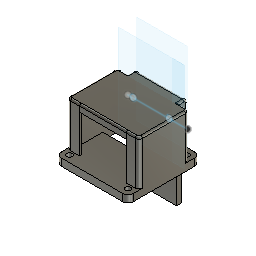
Optical Cube mk1 v4 (Autodesk Fusion 360 design; units mm, degrees)
Autodesk Fusion 360 part; units mm, degrees
note: some values were not read from the file. Set by a fixed rule: which sketch regions a step uses.
sketch "Sketch1" plane through (0, 0, 0) normal (0, 0, 1) x (1, 0, 0)
  line L0 (17, -20) -> (-17, -20)
  line L1 (-20, -17) -> (-20, 17)
  line L2 (-17, 20) -> (17, 20)
  line L3 (20, 17) -> (20, -17)
  line L4 (20, -20) -> (-20, 20) construction
  line L5 (-20, -20) -> (20, 20) construction
  arc A0 (-17, 20) -> (-20, 17) centre (-17, 17) ccw
  arc A1 (20, 17) -> (17, 20) centre (17, 17) ccw
  arc A2 (-20, -17) -> (-17, -20) centre (-17, -17) ccw
  arc A3 (17, -20) -> (20, -17) centre (17, -17) ccw
  dimension "d1" = 40
  dimension "d2" = 40
  dimension "d7" = 3
  dimension "d8" = 3
  dimension "d9" = 3
  dimension "d10" = 3
  constraint horizontal L0
  constraint perpendicular L0 L1
  constraint parallel L0 L2
  constraint parallel L1 L3
  constraint coincident L4 origin
  constraint coincident L5 origin
  constraint coincident L4.end L2
  constraint coincident L4.end L1
  constraint tangent L2 A0
  constraint tangent L1 A0
  constraint coincident L5.end L2
  constraint coincident L5.end L3
  constraint tangent L2 A1
  constraint tangent L3 A1
  constraint coincident L5.start L0
  constraint coincident L5.start L1
  constraint tangent L0 A2
  constraint tangent L1 A2
  constraint coincident L4.start L3
  constraint coincident L4.start L0
  constraint tangent L3 A3
  constraint tangent L0 A3
  measures "d1" distance of L4.end L5.end
  measures "d2" distance of L5.start L4.end
  measures "d7" radius of A0
  measures "d8" radius of A1
  measures "d9" radius of A2
  measures "d10" radius of A3
extrude "Extrude1" add sketch "Sketch1" along normal blind 4
sketch "Sketch3" plane through (0, 0, 4) normal (0, 0, 1) x (-1, 0, 0)
  arc A0 (20, 17) -> (17, 20) centre (17, 17) ccw
  line L0 (17, 20) -> (-17, 20)
  arc A1 (-17, 20) -> (-20, 17) centre (-17, 17) ccw
  line L1 (-20, 17) -> (-20, -17)
  arc A2 (-20, -17) -> (-17, -20) centre (-17, -17) ccw
  line L2 (-17, -20) -> (17, -20)
  arc A3 (17, -20) -> (20, -17) centre (17, -17) ccw
  line L3 (20, -17) -> (20, 17)
  circle A4 centre (16.2929, -16.2929) radius 1.5
  circle A5 centre (-16.2929, -16.2929) radius 1.5
  circle A6 centre (16.2929, 16.2929) radius 1.5
  circle A7 centre (-16.2929, 16.2929) radius 1.5
  line L4 (13.9939, -20) -> (13.9939, -14)
  line L5 (13.9939, -14) -> (20, -14)
  line L6 (20, 13.9693) -> (13.9939, 13.9693)
  line L7 (13.9939, 13.9693) -> (13.9939, 20)
  line L8 (-14.051, 20) -> (-14.051, 13.9693)
  line L9 (-14.051, 13.9693) -> (-20, 13.9693)
  line L10 (-20, -14) -> (-14.051, -14)
  line L11 (-14.051, -14) -> (-14.051, -20)
  line L12 (13.9939, -18.9303) -> (-14.051, -18.9303)
  line L13 (13.9939, 18.9046) -> (-14.051, 18.9046)
  line L14 (18.9336, 13.9693) -> (18.9336, -14)
  line L15 (-19, -14) -> (-19, 13.9693)
  line L16 (18.9336, -12.9942) -> (13, -12.9942)
  line L17 (13, -12.9942) -> (13, -18.9303)
  line L18 (17.9849, -12.9942) -> (17.9849, 13)
  line L19 (17.9849, 13) -> (13, 13)
  line L20 (13, 13) -> (13, 18)
  line L21 (13, 18) -> (-13, 18)
  line L22 (-13, 18) -> (-13, 13)
  line L23 (-13, 13) -> (-18, 13)
  line L24 (-18, 13) -> (-18, -13)
  line L25 (-18, -13) -> (-13, -13)
  line L26 (-13, -13) -> (-13, -18)
  line L27 (-13, -18) -> (13, -18)
  dimension "d13" = 3
  dimension "d15" = 3
  dimension "d17" = 3
  dimension "d19" = 3
  constraint coincident L2 L4.start
  constraint perpendicular L2 L4
  constraint coincident L3 L5.end
  constraint perpendicular L3 L5
  constraint coincident L3 L6.start
  constraint perpendicular L3 L6
  constraint coincident L0 L7.end
  constraint perpendicular L0 L7
  constraint coincident L0 L8.start
  constraint perpendicular L0 L8
  constraint coincident L1 L9.end
  constraint perpendicular L1 L9
  constraint coincident L1 L10.start
  constraint perpendicular L1 L10
  constraint coincident L2 L11.end
  constraint perpendicular L2 L11
  constraint coincident L4 L12.start
  constraint coincident L11 L12.end
  constraint perpendicular L11 L12
  constraint coincident L7 L13.start
  constraint coincident L8 L13.end
  constraint perpendicular L8 L13
  constraint coincident L6 L14.start
  constraint coincident L5 L14.end
  constraint perpendicular L5 L14
  constraint coincident L10 L15.start
  constraint coincident L9 L15.end
  constraint perpendicular L9 L15
  constraint coincident L14 L16.start
  constraint perpendicular L14 L16
  constraint coincident L12 L17.end
  constraint perpendicular L12 L17
  constraint coincident L16 L18.start
  constraint perpendicular L16 L18
  constraint perpendicular L18 L19
  constraint perpendicular L13 L20
  constraint perpendicular L8 L21
  constraint perpendicular L21 L22
  constraint perpendicular L22 L23
  constraint perpendicular L9 L24
  constraint perpendicular L24 L25
  constraint perpendicular L25 L26
  constraint coincident L17 L27.end
  constraint perpendicular L17 L27
  measures "d13" diameter of A4
  measures "d15" diameter of A5
  measures "d17" diameter of A6
  measures "d19" diameter of A7
extrude "Extrude2" add sketch "Sketch3" along normal blind 50 contours L6 L7 L8 L9 L10 L11 L12 L13 L14 L15 L16 L17 L18 L19 L20 L21 L22 L23 L24 L25 L26 L27 | L4 L5 L12 L14 L16 L17
extrude "Extrude4" cut sketch "Sketch3" against normal blind 42 contours A5
extrude "Extrude5" cut sketch "Sketch3" against normal blind 14 contours A4
extrude "Extrude6" cut sketch "Sketch3" against normal blind 15 contours A6
extrude "Extrude7" cut sketch "Sketch3" against normal blind 15 contours A7
extrude "Extrude8" add sketch "Sketch3" along normal blind 50 contours L16 L17 L18 L19 L20 L21 L22 L23 L24 L25 L26 L27
sketch "Sketch4" plane through (0, 0, 0) normal (0, 0, -1) x (1, 0, 0)
  circle A0 centre (16.2929, 16.2929) radius 1.5
  circle A1 centre (-16.2929, 16.2929) radius 1.5
  circle A2 centre (-16.2929, -16.2929) radius 1.5
  circle A3 centre (16.2929, -16.2929) radius 1.5
  arc A4 (-17, 20) -> (-20, 17) centre (-17, 17) ccw
  line L0 (-20, 17) -> (-20, -17)
  arc A5 (-20, -17) -> (-17, -20) centre (-17, -17) ccw
  line L1 (-17, -20) -> (17, -20)
  arc A6 (17, -20) -> (20, -17) centre (17, -17) ccw
  line L2 (20, -17) -> (20, 17)
  arc A7 (20, 17) -> (17, 20) centre (17, 17) ccw
  line L3 (17, 20) -> (-17, 20)
  line L4 (12, -18) -> (12, -13)
  line L5 (12, -13) -> (18, -13)
  line L6 (18, -13) -> (18, 13)
  line L7 (18, 13) -> (13, 13)
  line L8 (13, 13) -> (13, 18)
  line L9 (13, 18) -> (-13, 18)
  line L10 (-13, 18) -> (-13, 13)
  line L11 (-13, 13) -> (-18, 13)
  line L12 (-18, 13) -> (-18, -13)
  line L13 (-18, -13) -> (-13, -13)
  line L14 (-13, -13) -> (-13, -18)
  line L15 (-13, -18) -> (12, -18)
  constraint vertical L4
  constraint perpendicular L4 L5
  constraint perpendicular L5 L6
  constraint perpendicular L6 L7
  constraint perpendicular L7 L8
  constraint perpendicular L8 L9
  constraint perpendicular L9 L10
  constraint perpendicular L10 L11
  constraint perpendicular L11 L12
  constraint perpendicular L0 L13
  constraint perpendicular L13 L14
  constraint perpendicular L4 L15
extrude "Extrude9" cut sketch "Sketch4" against normal blind 50 contours L4 L5 L6 L7 L8 L9 L10 L11 L12 L13 L14 L15
sketch "Sketch5" plane through (-18, 0, 0) normal (1, 0, 0) x (0, 1, 0)
  line L0 (-13, 0) -> (13, 0)
  line L1 (13, 0) -> (13, 50)
  line L2 (13, 50) -> (-13, 50)
  line L3 (-13, 50) -> (-13, 0)
  line L4 (13, 0) -> (11, 0)
  line L5 (11, 0) -> (11, 50)
  line L6 (11, 50) -> (13, 50)
  line L7 (13, 50) -> (13, 0)
  dimension "d36" = 2
  dimension "d37" = 50
  constraint horizontal L4
  constraint vertical L5
  constraint horizontal L6
  constraint vertical L7
  constraint coincident L0.end L1.start
  measures "d36" distance of L0.end L4.end
  measures "d37" distance of L0.end L1.end
extrude "Extrude10" cut sketch "Sketch5" against normal blind 0.3 contours L0 L1 L2 L4 L5 L6 L7
sketch "Sketch6" plane through (18, 0, 0) normal (-1, 0, 0) x (0, -1, 0)
  line L0 (-13, 0) -> (13, 0)
  line L1 (13, 0) -> (13, 50)
  line L2 (13, 50) -> (-13, 50)
  line L3 (-13, 50) -> (-13, 0)
  line L4 (-13, 0) -> (-11, 0)
  line L5 (-11, 0) -> (-11, 50)
  line L6 (-11, 50) -> (-13, 50)
  line L7 (-13, 50) -> (-13, 0)
  dimension "d40" = 2
  dimension "d41" = 50
  constraint horizontal L4
  constraint vertical L5
  constraint horizontal L6
  constraint vertical L7
  constraint coincident L0.start L3.end
  measures "d40" distance of L0.start L4.end
  measures "d41" distance of L0.start L2.end
extrude "Extrude11" cut sketch "Sketch6" against normal blind 0.3 contours L0 L2 L3 L4 L5 L6 L7
sketch "Sketch7" plane through (-13.9939, 0, 0) normal (-1, 0, 0) x (0, -1, 0)
  line L0 (-18.9303, 4) -> (-14, 4)
  line L1 (-14, 4) -> (-14, 54)
  line L2 (-14, 54) -> (-18.9303, 54)
  line L3 (-18.9303, 54) -> (-18.9303, 4)
  line L4 (-18.9303, 54) -> (-14, 54)
  line L5 (-14, 54) -> (-14, 14)
  line L6 (-14, 14) -> (-18.9303, 14)
  line L7 (-18.9303, 14) -> (-18.9303, 54)
  constraint horizontal L4
  constraint vertical L5
  constraint horizontal L6
  constraint vertical L7
  constraint coincident L1 L5.end
  constraint coincident L2.end L3.start
extrude "Extrude12" add sketch "Sketch7" against normal blind 28 contours L1 L2 L3 L4 L5 L6 L7
sketch "Sketch9" plane through (0, 18.9303, 0) normal (0, 1, 0) x (-1, 0, 0)
  line L0 (-14.051, 4) -> (13.9939, 4)
  line L1 (13.9939, 4) -> (13.9939, 54)
  line L2 (13.9939, 54) -> (-14.051, 54)
  line L3 (-14.051, 54) -> (-14.051, 4)
  line L4 (18.9939, 14) -> (-14.051, 14)
  constraint coincident L3 L4.end
  constraint perpendicular L3 L4
sketch "Sketch11" plane through (14.051, 0, 0) normal (1, 0, 0) x (0, 1, 0)
  line L0 (14, 4) -> (18.9303, 4)
  line L1 (18.9303, 4) -> (18.9303, 54)
  line L2 (18.9303, 54) -> (14, 54)
  line L3 (14, 54) -> (14, 4)
  line L4 (14, 54) -> (18.9303, 54)
  line L5 (18.9303, 54) -> (18.9303, 13.913)
  line L6 (18.9303, 13.913) -> (14, 13.913)
  line L7 (14, 13.913) -> (14, 54)
  constraint horizontal L4
  constraint vertical L5
  constraint horizontal L6
  constraint vertical L7
  constraint coincident L1 L5.end
  constraint coincident L2.end L3.start
extrude "Extrude13" add sketch "Sketch11" along normal blind 5 contours L1 L2 L3 L4 L5 L6 L7
sketch "Sketch12" plane through (0, -18, 0) normal (0, 1, 0) x (-1, 0, 0)
  line L0 (-13, 0) -> (13, 0)
  line L1 (13, 0) -> (13, 50)
  line L2 (13, 50) -> (-13, 50)
  line L3 (-13, 50) -> (-13, 0)
  line L4 (-13, 50) -> (13, 50)
  line L5 (13, 50) -> (13, -6)
  line L6 (13, -6) -> (-13, -6)
  line L7 (-13, -6) -> (-13, 50)
  constraint horizontal L4
  constraint vertical L5
  constraint horizontal L6
  constraint vertical L7
  constraint coincident L2.end L3.start
extrude "Extrude14" cut sketch "Sketch12" against normal blind 13 contours L0 L1 L2 L3 L4 L5 L7
sketch "Sketch13" plane through (0, 13, 0) normal (0, -1, 0) x (1, 0, 0)
  line L0 (12, 0) -> (18.3, 0)
  line L1 (18.3, 0) -> (18.3, 50)
  line L2 (18.3, 50) -> (12, 50)
  line L3 (12, 50) -> (12, 0)
extrude "Extrude15" add 1 faces at (-13, 15, 4.6667) along direction (1, 0, 0) blind 26
extrude "Extrude16" cut 1 faces at (19.051, 15.6434, 40.6377) along direction (-1, 0, 0) blind 5
sketch "Sketch14" plane through (14.051, 0, 0) normal (1, 0, 0) x (0, 1, 0)
  line L0 (14, 54) -> (14, 4)
  line L1 (14, 4) -> (18.9303, 4)
  line L2 (18.9303, 4) -> (18.9303, 54)
  line L3 (18.9303, 54) -> (14, 54)
  line L4 (18.9303, 54) -> (14, 54)
  line L5 (14, 54) -> (14, 35)
  line L6 (14, 35) -> (18.9303, 35)
  line L7 (18.9303, 35) -> (18.9303, 54)
  constraint horizontal L4
  constraint vertical L5
  constraint horizontal L6
  constraint vertical L7
  constraint coincident L0 L5.end
  constraint coincident L2.end L3.start
extrude "Extrude17" add sketch "Sketch14" along normal blind 5 contours L0 L2 L3 L4 L5 L6 L7
sketch "Sketch15" plane through (-13.9939, 0, 0) normal (-1, 0, 0) x (0, -1, 0)
  line L0 (-18.9303, 54) -> (-18.9303, 4)
  line L1 (-18.9303, 4) -> (-14, 4)
  line L2 (-14, 4) -> (-14, 54)
  line L3 (-14, 54) -> (-18.9303, 54)
  line L4 (-18.9303, 54) -> (-14, 54)
  line L5 (-14, 54) -> (-14, 35)
  line L6 (-14, 35) -> (-18.9303, 35)
  line L7 (-18.9303, 35) -> (-18.9303, 54)
  constraint horizontal L4
  constraint vertical L5
  constraint horizontal L6
  constraint vertical L7
  constraint coincident L2 L5.end
  constraint coincident L0.start L3.end
extrude "Extrude18" add sketch "Sketch15" along normal blind 5 contours L0 L2 L3 L4 L5 L6 L7
sketch "Sketch16" plane through (0, 13, 0) normal (0, -1, 0) x (1, 0, 0)
  line L0 (-18.3, 0) -> (18.3, 0)
  line L1 (18.3, 0) -> (18.3, 50)
  line L2 (18.3, 50) -> (-18.3, 50)
  line L3 (-18.3, 50) -> (-18.3, 0)
  circle A0 centre (9.8744, 20.0869) radius 1.5
  circle A1 centre (-10.1256, 20.0869) radius 1.5
  dimension "d61" = 3
  dimension "d62" = 3
  dimension "d93" = 20
  measures "d61" diameter of A0
  measures "d62" diameter of A1
  measures "d93" distance of A0.centre A1.centre
extrude "Extrude19" cut sketch "Sketch16" against normal blind 12 contours A0 | A1
extrude "Extrude20" add 1 faces at (-13.9939, -15.6144, 37.3333) along direction (-1, 0, 0) blind 5
extrude "Extrude21" add 1 faces at (14.051, -17.2595, 37.3333) along direction (1, 0, 0) blind 5
sketch "Sketch17" plane through (19.051, 0, 0) normal (1, 0, 0) x (0, 1, 0)
  line L0 (-18.9046, 4) -> (-13.9693, 4)
  line L1 (-13.9693, 4) -> (-13.9693, 54)
  line L2 (-13.9693, 54) -> (-18.9046, 54)
  line L3 (-18.9046, 54) -> (-18.9046, 4)
  line L4 (-18.9046, 34.9752) -> (-13.9693, 34.9752)
  line L5 (-13.9693, 34.9752) -> (-13.9693, 4)
  line L6 (-13.9693, 4) -> (-18.9046, 4)
  line L7 (-18.9046, 4) -> (-18.9046, 34.9752)
  constraint horizontal L4
  constraint vertical L5
  constraint horizontal L6
  constraint vertical L7
  constraint coincident L0.end L1.start
  constraint coincident L3 L4.start
extrude "Extrude22" cut sketch "Sketch17" against normal blind 8 contours L0 L1 L3 L4 L5 L6 L7
sketch "Sketch18" plane through (-18.9939, 0, 0) normal (-1, 0, 0) x (0, -1, 0)
  line L0 (13.9693, 4) -> (18.9046, 4)
  line L1 (18.9046, 4) -> (18.9046, 54)
  line L2 (18.9046, 54) -> (13.9693, 54)
  line L3 (13.9693, 54) -> (13.9693, 4)
  line L4 (18.9046, 4) -> (13.9693, 4)
  line L5 (13.9693, 4) -> (13.9693, 35.0999)
  line L6 (13.9693, 35.0999) -> (18.9046, 35.0999)
  line L7 (18.9046, 35.0999) -> (18.9046, 4)
  constraint horizontal L4
  constraint vertical L5
  constraint horizontal L6
  constraint vertical L7
  constraint coincident L3 L5.end
  constraint coincident L0.end L1.start
extrude "Extrude23" cut sketch "Sketch18" against normal blind 6 contours L0 L1 L3 L4 L5 L6 L7
sketch "Sketch19" plane through (13, 0, 0) normal (-1, 0, 0) x (0, -1, 0)
  line L0 (13.9693, 34.9752) -> (18.9046, 34.9752)
  line L1 (18.9046, 34.9752) -> (18.9046, 50)
  line L2 (18.9046, 50) -> (13, 50)
  line L3 (13, 50) -> (13, 0)
  line L4 (13, 0) -> (20, 0)
  line L5 (20, 0) -> (20, 4)
  line L6 (20, 4) -> (13.9693, 4)
  line L7 (13.9693, 4) -> (13.9693, 34.9752)
  line L8 (20, 0) -> (13, 0)
  line L9 (13, 0) -> (13, 4)
  line L10 (13, 4) -> (20, 4)
  line L11 (20, 4) -> (20, 0)
  constraint horizontal L8
  constraint vertical L9
  constraint horizontal L10
  constraint vertical L11
  constraint coincident L3 L9.end
  constraint coincident L4.end L5.start
extrude "Extrude24" add sketch "Sketch19" along normal blind 26 contours L3 L4 L5 L6 L8 L9 L10 L11
sketch "Sketch20" plane through (0, -13, 0) normal (0, 1, 0) x (-1, 0, 0)
  line L0 (-18, 0) -> (18, 0)
  line L1 (18, 0) -> (18, 50)
  line L2 (18, 50) -> (13, 50)
  line L3 (13, 50) -> (13, 4)
  line L4 (13, 4) -> (-13, 4)
  line L5 (-13, 4) -> (-13, 50)
  line L6 (-13, 50) -> (-18, 50)
  line L7 (-18, 50) -> (-18, 0)
  line L8 (18, 0) -> (-18, 0)
  line L9 (-18, 0) -> (-18, 4)
  line L10 (-18, 4) -> (18, 4)
  line L11 (18, 4) -> (18, 0)
  constraint horizontal L8
  constraint vertical L9
  constraint horizontal L10
  constraint vertical L11
  constraint coincident L7 L9.end
  constraint coincident L0.end L1.start
extrude "Extrude25" add sketch "Sketch20" along normal blind 17 contours L0 L1 L4 L7 L8 L9 L10 L11
sketch "Sketch21" plane through (0, 4, 0) normal (0, 1, 0) x (-1, 0, 0)
  line L0 (18, 4) -> (-18, 4)
  line L1 (-18, 4) -> (-18, 0)
  line L2 (-18, 0) -> (18, 0)
  line L3 (18, 0) -> (18, 4)
  line L4 (-18, 4) -> (-13, 4)
  line L5 (-13, 4) -> (-13, 0)
  line L6 (-13, 0) -> (-18, 0)
  line L7 (-18, 0) -> (-18, 4)
  line L8 (18, 4) -> (13, 4)
  line L9 (13, 4) -> (13, 0)
  line L10 (13, 0) -> (18, 0)
  line L11 (18, 0) -> (18, 4)
  constraint horizontal L4
  constraint vertical L5
  constraint horizontal L6
  constraint vertical L7
  constraint coincident L2 L5.end
  constraint coincident L0.end L1.start
  constraint horizontal L8
  constraint vertical L9
  constraint horizontal L10
  constraint vertical L11
  constraint coincident L2 L9.end
  constraint coincident L0.start L3.end
extrude "Extrude26" add sketch "Sketch21" along normal blind 7 contours L0 L2 L3 L8 L9 L10 L11 | L0 L1 L2 L4 L5 L6 L7
extrude "Extrude27" add 1 faces at (13, 8.6667, 2.6667) along direction (-1, 0, 0) blind 5
extrude "Extrude28" add 1 faces at (-13, 8.6667, 2.6667) along direction (1, 0, 0) blind 5
extrude "Extrude29" cut 1 faces at (8, 8.6667, 2.6667) along direction (1, 0, 0) blind 10
extrude "Extrude30" cut 1 faces at (-8, 8.6667, 2.6667) along direction (-1, 0, 0) blind 10
extrude "Extrude31" add 1 faces at (19, 4.6769, 24.6584) along direction (1, 0, 0) blind 1
extrude "Extrude32" add 1 faces at (-18.9336, -4.6462, 24.7) along direction (-1, 0, 0) blind 1
move_face "OffsetFaces1" offset 3 1 faces at (-4.3333, 3, 50)
move_face "OffsetFaces2" offset -1 1 faces at (-4.3333, 3, 47)
extrude "Extrude33" add 1 faces at (-18.9939, 17.2869, 41.3333) along direction (-1, 0, 0) blind 1
extrude "Extrude34" add 1 faces at (-18.9939, -15.6144, 41.3999) along direction (-1, 0, 0) blind 1
extrude "Extrude35" add 1 faces at (19.051, -17.2595, 41.3168) along direction (1, 0, 0) blind 1
extrude "Extrude36" add 1 faces at (19.051, 15.6434, 47.6667) along direction (1, 0, 0) blind 1
fillet "Fillet1" radius 3 1 edges at (20.051, 18.9303, 44.5)
fillet "Fillet2" radius 3 1 edges at (-19.9939, 18.9303, 44.5)
fillet "Fillet3" radius 3 1 edges at (-19.9939, -18.9046, 44.5499)
fillet "Fillet4" radius 3 1 edges at (20.051, -18.9046, 44.4876)
move_face "OffsetFaces3" offset 8 1 faces at (-4.3333, 3, 48)
move_face "OffsetFaces4" offset -10 1 faces at (6.6888, -4.6462, 54)
sketch "Sketch22" plane through (0, 0, 0) normal (0, 0, -1) x (1, 0, 0)
  line L0 (-18, -11) -> (-18, -4)
  line L1 (-18, -4) -> (18, -4)
  line L2 (18, -4) -> (18, -11)
  line L3 (18, -11) -> (18.3, -11)
  line L4 (18.3, -11) -> (18.3, -13)
  line L5 (18.3, -13) -> (-18.3, -13)
  line L6 (-18.3, -13) -> (-18.3, -11)
  line L7 (-18.3, -11) -> (-18, -11)
  circle A0 centre (16.2929, 16.2929) radius 1.5
  circle A1 centre (-16.2929, 16.2929) radius 1.5
  circle A2 centre (-16.2929, -16.2929) radius 1.5
  circle A3 centre (16.2929, -16.2929) radius 1.5
  line L8 (17, 20) -> (-17, 20)
  arc A4 (-17, 20) -> (-20, 17) centre (-17, 17) ccw
  line L9 (-20, 17) -> (-20, -17)
  arc A5 (-20, -17) -> (-17, -20) centre (-17, -17) ccw
  line L10 (-17, -20) -> (17, -20)
  arc A6 (17, -20) -> (20, -17) centre (17, -17) ccw
  line L11 (20, -17) -> (20, 17)
  arc A7 (20, 17) -> (17, 20) centre (17, 17) ccw
  line L12 (14, -13) -> (-14, -13)
  line L13 (-14, -13) -> (-14, -16)
  line L14 (-14, -16) -> (14, -16)
  line L15 (14, -16) -> (14, -13)
  constraint horizontal L12
  constraint vertical L13
  constraint horizontal L14
  constraint vertical L15
  constraint coincident L5 L12.start
extrude "Extrude37" add sketch "Sketch22" along normal blind 20 contours L5 L12 L13 L14 L15
extrude "Extrude38" add 1 faces at (-4.3333, 3, 40) along direction (0, 0, -1) blind 11
move_face "OffsetFaces5" offset -5 1 faces at (6.6888, -4.6462, 44)
move_face "OffsetFaces6" offset 6.5 4 faces at (-16.9939, 16.2869, 35) (17.051, 16.2869, 35) (16.7007, -16.2595, 34.9752) (-16.6626, -16.2595, 35.0999)
extrude "Extrude39" cut 1 faces at (6.6888, -4.6462, 39) along direction (0, 0, -1) blind 6
extrude "Extrude40" add 1 faces at (-4.3333, 3, 29) along direction (0, 0, -1) blind 4
extrude "Extrude41" cut 1 faces at (6.6888, -4.6462, 33) along direction (0, 0, -1) blind 4
extrude "Extrude42" cut 1 faces at (17.051, 16.2869, 28.5) along direction (0, 0, 1) blind 5
extrude "Extrude43" cut 1 faces at (-16.9939, 16.2869, 28.5) along direction (0, 0, 1) blind 7
extrude "Extrude44" cut 1 faces at (16.7007, -16.2595, 28.4752) along direction (0, 0, 1) blind 8
extrude "Extrude45" cut 1 faces at (-16.6626, -16.2595, 28.5999) along direction (0, 0, 1) blind 7
fillet "Fillet5" radius 2 1 edges at (-19.9336, -13.9693, 16.5)
fillet "Fillet6" radius 2 1 edges at (-19.9336, 14, 16.5)
fillet "Fillet7" radius 2 1 edges at (20, 14, 16.5)
fillet "Fillet8" radius 2 1 edges at (20, -13.9693, 16.5)
move_face "OffsetFaces7" offset -5 1 faces at (-4.3333, -18.9046, 26.3333)
fillet "Fillet9" radius 2 1 edges at (0.0285, 18.9303, 29)
fillet "Fillet10" radius 1 11 edges at (15.5, -13.9693, 29) (19.4142, -13.3835, 29) (20, 0.0153, 29) (19.4142, 13.4142, 29) (16.0255, 14, 29) (0, -13.9046, 29) (-15.9637, 14, 29) (-19.3478, 13.4142, 29) (-19.9336, 0.0153, 29) (-19.3478, -13.3835, 29) (-15.4668, -13.9693, 29)
fillet "Fillet11" radius 1 6 edges at (-13.9939, 18.9303, 15.5) (-13.9939, 18.3445, 28.4142) (-13.9939, 14.9652, 29) (14.051, 14.9652, 29) (14.051, 18.3445, 28.4142) (14.051, 18.9303, 15.5)
